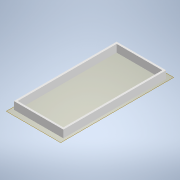
# Autodesk Inventor part: Mid
Saved by Autodesk Inventor 2022 (Build 260153000, 153)
## iProperties
Created: 2023-01-03
Part Number: Mid
Material: Generic
Document SubType Name: Modeling
Designer: karpova
Density: 1 g/cm^3
Appearance: Default
Author: karpova
Autodesk Inventor part; units mm, degrees
ref_plane "YZ Plane" through (0, 0, 0) normal (1, 0, 0) x (0, 1, 0)
ref_plane "XZ Plane" through (0, 0, 0) normal (0, 1, 0) x (-1, 0, 0)
ref_plane "XY Plane" through (0, 0, 0) normal (0, 0, 1) x (1, 0, 0)
ref_plane "Work Plane1" through (47.167, -27.5147, -55.5227) normal (0, 1, 0) x (1, 0, 0)
sketch "Sketch1" plane through (47.167, -27.5147, -55.5227) normal (0, 1, 0) x (1, 0, 0)
  line L0 (-26, -54) -> (26, -54) projected
  line L1 (-26, 54) -> (-26, -54) projected
  line L2 (-26, -54) -> (26, -54) projected
  line L3 (26, -54) -> (26, 54) projected
  line L4 (26, 54) -> (-26, 54) projected
  line L5 (25.5, 53.5) -> (25.5, -53.5) projected
  line L6 (25.5, -53.5) -> (-25.5, -53.5) projected
  line L7 (-25.5, -53.5) -> (-25.5, 53.5) projected
  line L8 (-25.5, 53.5) -> (25.5, 53.5) projected
  line L9 (-24.5, -52.5) -> (24.5, -52.5) projected
  line L10 (24.5, -52.5) -> (24.5, 52.5) projected
  line L11 (24.5, 52.5) -> (-24.5, 52.5) projected
  line L12 (-24.5, 52.5) -> (-24.5, -52.5) projected
  line L13 (-24, -52) -> (-24, 52) projected
  line L14 (-24, 52) -> (24, 52) projected
  line L15 (24, 52) -> (24, -52) projected
  line L16 (24, -52) -> (-24, -52) projected
  point P0 (-47.167, -55.5227)
extrude "Extrusion1" add sketch "Sketch1" along normal blind 7.9375 contours L1 L4 L3 L0 | L5 L6 L7 L8 | L12 L11 L10 L9
sketch "Sketch2" plane through (47.167, -27.5147, -55.5227) normal (0, -1, 0) x (1, 0, 0)
  line L0 (-26, 54) -> (-26, -54) projected
  line L1 (-26, -54) -> (26, -54) projected
  line L2 (26, -54) -> (26, 54) projected
  line L3 (26, 54) -> (-26, 54) projected
  line L4 (-25, -53) -> (-25, 53) construction
  line L5 (-25, 53) -> (25, 53) construction
  line L6 (25, 53) -> (25, -53) construction
  line L7 (25, -53) -> (-25, -53) construction
  line L8 (-25.5, -53.5) -> (-25.5, 53.5)
  line L9 (-25.5, 53.5) -> (25.5, 53.5)
  line L10 (25.5, 53.5) -> (25.5, -53.5)
  line L11 (25.5, -53.5) -> (-25.5, -53.5)
  line L12 (-24.5, 52.5) -> (-24.5, -52.5)
  line L13 (-24.5, -52.5) -> (24.5, -52.5)
  line L14 (24.5, -52.5) -> (24.5, 52.5)
  line L15 (24.5, 52.5) -> (-24.5, 52.5)
  point P0 (-47.167, 55.5227)
  dimension "d2" = 1
  dimension "d3" = 1
  constraints: 24 end point, 10 other
  measures "d2" distance between parallel lines of L0 L4
  measures "d3" distance between parallel lines of L12 L8
extrude "Extrusion2" cut sketch "Sketch2" against normal blind 0.5 contours L8 L9 L10 L11
chamfer "Chamfer1" distance 0.25 angle 45 8 edges at (71.667, -27.0147, -55.5227) (47.167, -27.0147, -3.0227) (72.667, -27.0147, -55.5227) (47.167, -27.0147, -2.0227) (21.667, -27.0147, -55.5227) (22.667, -27.0147, -55.5227) (47.167, -27.0147, -108.0227) (47.167, -27.0147, -109.0227)
sketch "Sketch3" plane through (47.167, -19.5772, -55.5227) normal (0, 1, 0) x (1, 0, 0)
  line L0 (8, 26) -> (8, 24) projected
  line L1 (12, 24) -> (8, 24) projected
  line L2 (12, 48) -> (12, 24) projected
  line L3 (-12, 48) -> (12, 48) projected
  line L4 (-12, 24) -> (-12, 48) projected
  line L5 (-8, 24) -> (-12, 24) projected
  line L6 (-8, 24) -> (-8, 26) projected
  line L7 (-10, 26) -> (-8, 26) projected
  line L8 (-10, 46) -> (-10, 26) projected
  line L9 (10, 46) -> (-10, 46) projected
  line L10 (10, 26) -> (10, 46) projected
  line L11 (8, 26) -> (10, 26) projected
  line L12 (24, 52) -> (24, -52) projected
  line L13 (-24, 52) -> (24, 52) projected
  line L14 (-24, -52) -> (-24, 52) projected
  line L15 (24, -52) -> (-24, -52) projected
  line L16 (-8, 24) -> (8, 24)
  line L17 (8, 24) -> (8, 26)
  line L18 (8, 26) -> (-8, 26)
  line L19 (-8, 26) -> (-8, 24)
  point P0 (-47.167, -55.5227)
  constraints: 8 end point, 2 parallel, 1 horizontal, 1 perpendicular
extrude "Extrusion3" add sketch "Sketch3" against normal blind 2 contours L11 L10 L9 L8 L7 L6 L5 L4 L3 L2 L1 L0 | L0 L16 L6 L18 | L12 L15 L14 L13
sketch "Sketch4" plane through (47.167, -19.5772, -55.5227) normal (0, 1, 0) x (1, 0, 0)
  line L0 (10, 26) -> (-10, 26) projected
  line L1 (-10, 26) -> (-10, 46) projected
  line L2 (-10, 46) -> (10, 46) projected
  line L3 (10, 46) -> (10, 26) projected
  line L4 (-26, -54) -> (26, -54) projected
  line L5 (26, -54) -> (26, 54) projected
  line L6 (26, 54) -> (-26, 54) projected
  line L7 (-26, 54) -> (-26, -54) projected
  line L8 (-12, 48) -> (-12, 24)
  line L9 (-12, 24) -> (12, 24)
  line L10 (12, 24) -> (12, 48)
  line L11 (12, 48) -> (-12, 48)
  point P0 (-47.167, -55.5227)
  dimension "d11" = 2
  constraints: 8 end point, 3 other
  measures "d11" distance between parallel lines of L1 L8
extrude "Extrusion4" add sketch "Sketch4" along normal blind 5.175 contours L11 L10 L9 L8
fillet "Fillet1" radius 4 4 edges at (47.167, -19.5772, -79.5227) (59.167, -19.5772, -91.5227) (47.167, -19.5772, -103.5227) (35.167, -19.5772, -91.5227)
equation "\"d2\" = 0.5 * outerShellThickness"
equation "\"d3\" = 0.5 * outerShellThickness"
equation "\"d9\" = outerShellThickness"
equation "\"d11\" = outerShellThickness"
equation "\"outerShellThickness\" = 2"
body "Solid1"
